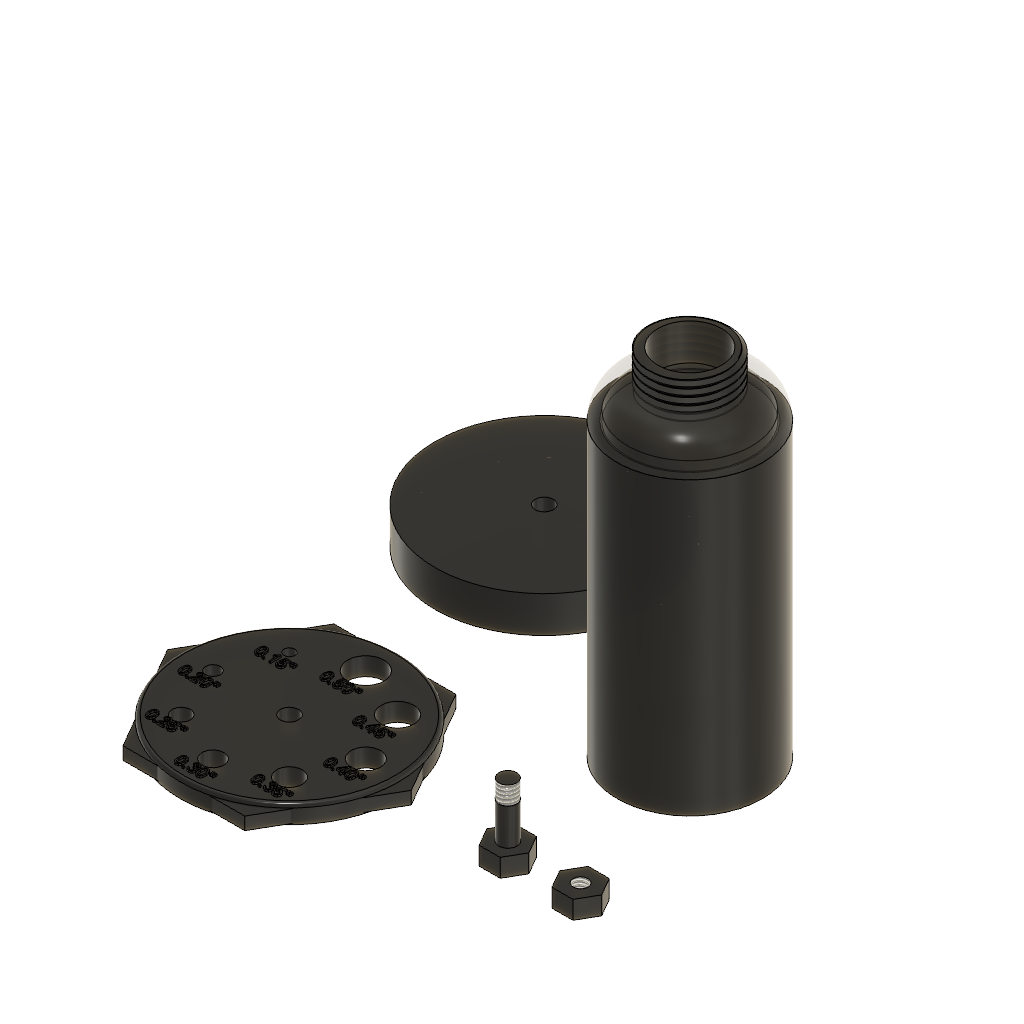
PillFilter Proof of Concept (Autodesk Fusion 360 design; units mm, degrees)
Autodesk Fusion 360 part; units mm, degrees
note: some values were not read from the file. Set by a fixed rule: the direction of a hole.
sketch "Filter Body" plane through (0, 0, 0) normal (0, 0, 1) x (1, 0, 0)
  circle A0 centre (0, 0) radius 38.1
  constraint coincident A0.centre origin
extrude "Extrude3" add sketch "Filter Body" along normal blind 6.35 makes body 1
hole "Hole5" at (0, 0, 6.35) direction (0, 0, -1) diameter 6.35 end through all bodies 1
sketch ".5\" Hole" plane through (0, 0, 6.35) normal (0, 0, 1) x (-1, 0, 0)
  circle A0 centre (0, 0) radius 3.175
  circle A1 centre (0, 0) radius 38.1
  circle A2 centre (0, -26.67) radius 6.35
  dimension "d27" = 12.7
  measures "d27" diameter of A2
sketch ".45\" Hole" plane through (0, 0, 6.35) normal (0, 0, 1) x (-1, 0, 0)
  circle A0 centre (-18.8585, -18.8585) radius 5.715
  dimension "d28" = 11.43
  measures "d28" diameter of A0
sketch ".4\" Hole" plane through (0, 0, 6.35) normal (0, 0, 1) x (-1, 0, 0)
  circle A0 centre (-26.67, 0) radius 5.08
  dimension "d29" = 10.16
  measures "d29" diameter of A0
sketch ".35\" Hole" plane through (0, 0, 6.35) normal (0, 0, 1) x (-1, 0, 0)
  circle A0 centre (-18.8585, 18.8585) radius 4.445
  dimension "d30" = 8.89
  measures "d30" diameter of A0
sketch "Lines (1.05\")" plane through (0, 0, 6.35) normal (0, 0, 1) x (1, 0, 0)
  line L0 (0, 0) -> (18.8585, 18.8585)
  line L1 (0, 0) -> (26.67, 0) construction
  line L2 (0, 0) -> (18.8585, -18.8585)
  line L3 (0, 0) -> (26.67, 0) construction
  line L4 (0, 0) -> (-18.8585, 18.8585)
  line L5 (0, 0) -> (-18.8585, -18.8585)
  line L6 (0, 0) -> (0, -26.67)
  line L7 (0, 0) -> (-26.67, 0)
  line L8 (0, 0) -> (0, 26.67)
  dimension "d31" = 45
  dimension "d32" = 26.67
  dimension "d33" = 45
  dimension "d34" = 26.67
  dimension "d36" = 26.67
  dimension "d37" = 26.67
  dimension "d38" = 26.67
  dimension "d39" = 26.67
  dimension "d45" = 26.67
  constraint horizontal L1
  constraint coincident L0.start L1.start
  constraint horizontal L3
  constraint perpendicular L0 L4
  constraint perpendicular L4 L5
  constraint perpendicular L1 L6
  constraint perpendicular L6 L7
  constraint perpendicular L3 L8
  measures "d31" angle of L0 L1
  measures "d32" distance of L0.start L0.end
  measures "d33" angle of L2 L3
  measures "d34" distance of L0.start L2.end
  measures "d36" distance of L0.start L4.end
  measures "d37" distance of L0.start L5.end
  measures "d38" distance of L0.start L6.end
  measures "d39" distance of L0.start L7.end
  measures "d45" distance of L0.start L8.end
sketch ".3\" Hole" plane through (0, 0, 6.35) normal (0, 0, 1) x (-1, 0, 0)
  circle A0 centre (0, 26.67) radius 3.81
  dimension "d41" = 7.62
  measures "d41" diameter of A0
sketch ".25\" Hole" plane through (0, 0, 6.35) normal (0, 0, 1) x (-1, 0, 0)
  circle A0 centre (18.8585, 18.8585) radius 3.175
  dimension "d42" = 6.35
  measures "d42" diameter of A0
sketch ".2\" Hole" plane through (0, 0, 6.35) normal (0, 0, 1) x (-1, 0, 0)
  circle A0 centre (26.67, 0) radius 2.54
  dimension "d43" = 5.08
  measures "d43" diameter of A0
sketch ".15\" Hole" plane through (0, 0, 6.35) normal (0, 0, 1) x (-1, 0, 0)
  circle A0 centre (18.8585, -18.8585) radius 1.905
  dimension "d44" = 3.81
  measures "d44" diameter of A0
hole "Hole6" at (0, 26.67, 6.35) direction (0, 0, -1) diameter 12.7 end through all bodies 1
hole "Hole7" at (18.8585, 18.8585, 6.35) direction (0, 0, -1) diameter 11.43 depth 12.7 tip angle 118 bodies 1
hole "Hole8" at (26.67, 0, 6.35) direction (0, 0, -1) diameter 10.16 end through all bodies 1
hole "Hole9" at (18.8585, -18.8585, 6.35) direction (0, 0, -1) diameter 8.89 depth 6.35 tip angle 118 bodies 1
hole "Hole10" at (0, -26.67, 6.35) direction (0, 0, -1) diameter 7.62 depth 6.35 tip angle 118 bodies 1
hole "Hole11" at (-18.8585, -18.8585, 6.35) direction (0, 0, -1) diameter 6.35 depth 6.35 tip angle 118 bodies 1
hole "Hole12" at (-26.67, 0, 6.35) direction (0, 0, -1) diameter 5.08 depth 6.35 tip angle 118 bodies 1
hole "Hole13" at (-18.8585, 18.8585, 6.35) direction (0, 0, -1) diameter 3.81 end through all bodies 1
sketch "Filter Backplate" plane through (0, 0, 0) normal (0, 0, 1) x (1, 0, 0)
  circle A0 centre (0, 88.9) radius 38.1
extrude "Extrude4" add sketch "Filter Backplate" along normal blind 6.35 separate body makes body 2
sketch "Backplate .5\" Hole" plane through (0, 0, 0) normal (0, 0, 1) x (1, 0, 0)
  circle A0 centre (0, 115.57) radius 6.35
  dimension "d71" = 12.7
  measures "d71" diameter of A0
hole "Hole14" at (0, 115.57, 0) direction (0, 0, 1) diameter 12.7 depth 12.7 tip angle 118 bodies 2
hole "Hole15" at (0, 88.9, 6.35) direction (0, 0, -1) diameter 6.35 end through all bodies 2
sketch "\"Text" plane through (0, 0, 6.35) normal (0, 0, 1) x (-1, 0, 0)
  line L0 (5.08, -16.51) -> (-5.08, -16.51) construction
  line L1 (-5.08, -16.51) -> (-5.08, -19.05) construction
  line L2 (-5.08, -19.05) -> (5.08, -19.05) construction
  line L3 (5.08, -19.05) -> (5.08, -16.51) construction
  line L4 (-15.2738, -8.7841) -> (-22.8759, -8.929) construction
  line L5 (-22.8759, -8.929) -> (-22.8262, -11.5359) construction
  line L6 (-22.8262, -11.5359) -> (-15.2241, -11.391) construction
  line L7 (-15.2241, -11.391) -> (-15.2738, -8.7841) construction
  line L8 (-22.86, 8.89) -> (-30.48, 8.89) construction
  line L9 (-30.48, 8.89) -> (-30.48, 6.35) construction
  line L10 (-30.48, 6.35) -> (-22.86, 6.35) construction
  line L11 (-22.86, 6.35) -> (-22.86, 8.89) construction
  line L12 (-15.24, 26.67) -> (-22.86, 26.67) construction
  line L13 (-22.86, 26.67) -> (-22.86, 24.13) construction
  line L14 (-22.86, 24.13) -> (-15.24, 24.13) construction
  line L15 (-15.24, 24.13) -> (-15.24, 26.67) construction
  line L16 (5.08, 34.29) -> (-5.08, 34.29) construction
  line L17 (-5.08, 34.29) -> (-5.08, 31.75) construction
  line L18 (-5.08, 31.75) -> (5.08, 31.75) construction
  line L19 (5.08, 31.75) -> (5.08, 34.29) construction
  line L20 (22.86, 25.4) -> (15.24, 25.4) construction
  line L21 (15.24, 25.4) -> (15.24, 22.86) construction
  line L22 (15.24, 22.86) -> (22.86, 22.86) construction
  line L23 (22.86, 22.86) -> (22.86, 25.4) construction
  line L24 (30.48, 6.35) -> (22.86, 6.35) construction
  line L25 (22.86, 6.35) -> (22.86, 3.81) construction
  line L26 (22.86, 3.81) -> (30.48, 3.81) construction
  line L27 (30.48, 3.81) -> (30.48, 6.35) construction
  line L28 (22.86, -12.7) -> (15.24, -12.7) construction
  line L29 (15.24, -12.7) -> (15.24, -15.24) construction
  line L30 (15.24, -15.24) -> (22.86, -15.24) construction
  line L31 (22.86, -15.24) -> (22.86, -12.7) construction
  dimension "d77" = 3.81
  dimension "d78" = 0
  dimension "d79" = 3.81
  dimension "d80" = 0
  dimension "d81" = 3.81
  dimension "d82" = 0
  dimension "d83" = 3.81
  dimension "d84" = 0
  dimension "d85" = 3.81
  dimension "d86" = 0
  dimension "d87" = 3.81
  dimension "d88" = 0
  dimension "d89" = 3.81
  dimension "d90" = 0
  dimension "d91" = 3.81
  dimension "d92" = 0
  text T0 "0.50\"" font "Arial" height 3.81 align centre middle in box 10.16 x 2.54 at (5.08, -16.51) x (-1, 0) y (0, -1) spacing 1 kerned
  text T1 "0.45\"" font "Arial" height 3.81 align centre middle in box 7.6035 x 2.6074 at (-15.2738, -8.7841) x (-0.999818, -0.019056) y (0.019056, -0.999818) spacing 1 kerned
  text T2 "0.40\"" font "Arial" height 3.81 align centre middle in box 7.62 x 2.54 at (-22.86, 8.89) x (-1, 0) y (0, -1) spacing 1 kerned
  text T3 "0.35\"" font "Arial" height 3.81 align centre middle in box 7.62 x 2.54 at (-15.24, 26.67) x (-1, 0) y (0, -1) spacing 1 kerned
  text T4 "0.30\"" font "Arial" height 3.81 align centre middle in box 10.16 x 2.54 at (5.08, 34.29) x (-1, 0) y (0, -1) spacing 1 kerned
  text T5 "0.25\"" font "Arial" height 3.81 align centre middle in box 7.62 x 2.54 at (22.86, 25.4) x (-1, 0) y (0, -1) spacing 1 kerned
  text T6 "0.20\"" font "Arial" height 3.81 align centre middle in box 7.62 x 2.54 at (30.48, 6.35) x (-1, 0) y (0, -1) spacing 1 kerned
  text T7 "0.15\"" font "Arial" height 3.81 align centre middle in box 7.62 x 2.54 at (22.86, -12.7) x (-1, 0) y (0, -1) spacing 1 kerned
extrude "Extrude5" add sketch "\"Text" along normal blind 0.635 text T0 T1 T2 T3 T4 T5 T6 T7 bodies 1
fillet "Fillet1" radius 1.27 1 edges at (-35.5217, -13.7775, 6.35) on bodies 1
sketch "Hex-Grip" plane through (0, 0, 0) normal (0, 0, 1) x (1, 0, 0)
  line L0 (-21.2638, 36.83) -> (-42.5276, 0)
  line L1 (-42.5276, 0) -> (-21.2638, -36.83)
  line L2 (-21.2638, -36.83) -> (21.2638, -36.83)
  line L3 (21.2638, -36.83) -> (42.5276, 0)
  line L4 (42.5276, 0) -> (21.2638, 36.83)
  line L5 (21.2638, 36.83) -> (-21.2638, 36.83)
  dimension "d97" = 36.83
  measures "d97" distance of origin L5
extrude "Extrude6" add sketch "Hex-Grip" along normal blind 4.445 separate body makes body 3
move_body "Move1" bodies 3 to x (1, 0, 0) y (0, 1, 0) z (0, 0, 1) at (0, 0, 0.3175)
sketch "Sketch24" plane through (0, 0, 4.7625) normal (0, 0, 1) x (-1, 0, 0)
  line L0 (-21.2638, -36.83) -> (21.2638, -36.83)
  line L1 (21.2638, -36.83) -> (42.5276, 0)
  line L2 (42.5276, 0) -> (21.2638, 36.83)
  line L3 (21.2638, 36.83) -> (-21.2638, 36.83)
  line L4 (-21.2638, 36.83) -> (-42.5276, 0)
  line L5 (-42.5276, 0) -> (-21.2638, -36.83)
hole "Hole16" at (0, 0, 4.7625) direction (0, 0, -1) diameter 67.31 depth 15.24 tip angle 118 bodies 3
sketch "Neck" plane through (0, 0, 0) normal (0, 0, -1) x (1, 0, 0)
  circle A0 centre (0, -88.9) radius 3.175
  circle A1 centre (0, -115.57) radius 6.35
  circle A2 centre (0, -88.9) radius 38.1
  circle A3 centre (0, -111.125) radius 15.875
  dimension "d103" = 31.75
  measures "d103" diameter of A3
extrude "Extrude7" add sketch "Neck" along normal blind 12.7 contours A3 bodies 2
move_body "Move2" bodies 2 to x (1, 0, 0) y (0, 1, 0) z (0, 0, 1) at (0, 0, 12.7)
sketch "Neck Receptacle" plane through (0, 0, 0) normal (0, 0, -1) x (1, 0, 0)
  circle A0 centre (0, -111.125) radius 13.335
hole "Hole17" at (0, 111.125, 0) direction (0, 0, 1) diameter 25.4 depth 12.7 tip angle 180 bodies 2
thread "Thread1" "ANSI Unified Screw Threads 1.125 1 1/8-10 UNS 1 1/8-10 UNS 2B" major diameter 28.575 minor diameter 26.0985 pitch 2.54 angle 60 modelled right hand crest width 0.7347 on face at (1.2645, 123.7619, 4.2333) crest through (-13.0493, 111.125, 0.635) on bodies 2
sketch "BottleBase" plane through (0, 0, 0) normal (0, 0, 1) x (1, 0, 0)
  circle A0 centre (76.2, 63.5) radius 25.4
  dimension "d111" = 50.8
  measures "d111" diameter of A0
extrude "Extrude8" add sketch "BottleBase" along normal blind 101.6 separate body makes body 4
hole "Hole18" at (76.2, 63.5, 101.6) direction (0, 0, -1) diameter 44.45 depth 98.425 tip angle 180 bodies 4
sketch "BottleShoulders" plane through (0, 0, 101.6) normal (0, 0, 1) x (-1, 0, 0)
  circle A0 centre (-76.2, -63.5) radius 22.225
  circle A1 centre (-76.2, -63.5) radius 25.4
  circle A2 centre (-76.2, -63.5) radius 25.4
  constraint concentric A0 A2
sketch "BottleShoulders (1)" plane through (0, 0, 101.6) normal (0, 0, 1) x (-1, 0, 0)
  circle A0 centre (-76.2, -63.5) radius 22.225
  circle A1 centre (-76.2, -63.5) radius 25.4
  circle A2 centre (-76.2, -63.5) radius 25.4
  constraint concentric A0 A2
extrude "Extrude10" add sketch "BottleShoulders (1)" along normal blind 12.7 separate body contours A0 | A1 A2 makes body 5
fillet "Fillet2" radius 12.7 1 edges at (99.8811, 72.685, 114.3) on bodies 5
shell "Shell1" thickness 3.175 removed faces 0 bodies 5
hole "Hole19" at (76.2, 63.5, 114.3) direction (0, 0, -1) diameter 25.4 depth 25.4 tip angle 180 bodies 5
hole "Hole20" at (76.2, 63.5, 104.775) direction (0, 0, -1) diameter 43.434 depth 25.4 tip angle 180 bodies 5
sketch "BottleNeck" plane through (0, 0, 101.6) normal (0, 0, 1) x (-1, 0, 0)
  circle A0 centre (-76.2, -63.5) radius 22.225
  circle A1 centre (-76.2, -63.5) radius 25.4
  circle A2 centre (-76.2, -63.5) radius 12.7
  dimension "d130" = 25.4
  constraint concentric A0 A2
  measures "d130" diameter of A2
extrude "Extrude11" add sketch "BottleNeck" along normal blind 12.7 separate body contours A2 makes body 6
move_body "Move3" bodies 6 to x (1, 0, 0) y (0, 1, 0) z (0, 0, 1) at (0, 0, 17.78)
move_body "Move4" bodies 6 to x (1, 0, 0) y (0, 1, 0) z (0, 0, 1) at (0, 0, -8.255)
thread "Thread2" "ANSI Unified Screw Threads 1.125 1 1/8-10 UNS 1 1/8-10 UNS 2A" major diameter 28.3667 minor diameter 25.5067 pitch 2.54 angle 60 modelled right hand crest width 0.3652 on face at (63.5631, 64.7645, 119.5917) crest through (62.0166, 63.5, 110.49) on bodies 6
hole "Hole21" at (76.2, 63.5, 123.825) direction (0, 0, -1) diameter 22.225 depth 25.4 tip angle 180 bodies 6
extrude "Extrude12" add 1 faces at (-13.0647, 104.1536, 19.05) along direction (0, 0, 1) blind 6.35 on bodies 2 bodies 2
sketch "BoltHead" plane through (0, 0, 0) normal (0, 0, 1) x (1, 0, 0)
  line L0 (72.5338, 6.35) -> (68.8677, 0)
  line L1 (68.8677, 0) -> (72.5338, -6.35)
  line L2 (72.5338, -6.35) -> (79.8662, -6.35)
  line L3 (79.8662, -6.35) -> (83.5324, 0)
  line L4 (83.5324, 0) -> (79.8662, 6.35)
  line L5 (79.8662, 6.35) -> (72.5338, 6.35)
  point P0 (76.2, 0)
  dimension "d146" = 6.35
  measures "d146" distance of P0 L5
extrude "Extrude13" add sketch "BoltHead" along normal blind 6.35 separate body makes body 7
sketch "BoltShank" plane through (0, 0, 6.35) normal (0, 0, 1) x (-1, 0, 0)
  line L0 (-79.8662, -6.35) -> (-72.5338, -6.35)
  line L1 (-72.5338, -6.35) -> (-68.8677, 0)
  line L2 (-68.8677, 0) -> (-72.5338, 6.35)
  line L3 (-72.5338, 6.35) -> (-79.8662, 6.35)
  line L4 (-79.8662, 6.35) -> (-83.5324, 0)
  line L5 (-83.5324, 0) -> (-79.8662, -6.35)
  circle A0 centre (-76.2, 0) radius 3.175
  dimension "d149" = 6.35
  measures "d149" diameter of A0
extrude "Extrude14" add sketch "BoltShank" along normal blind 12.7 contours A0 bodies 7
extrude "Extrude15" add 1 faces at (75.1887, 0.3119, 19.05) along direction (0, 0, 1) blind 6.35 separate body on bodies 7 makes body 8
thread "Thread3" "ANSI Unified Screw Threads 0.25 1/4-20 UNC 1/4-20 UNC 3A" major diameter 6.2484 minor diameter 4.8387 pitch 1.27 angle 60 resizes the face on face at (73.0408, 0.3161, 23.2833) on bodies 8
sketch "Nut" plane through (0, 0, 0) normal (0, 0, 1) x (1, 0, 0)
  line L0 (97.9338, 6.35) -> (94.2677, 0)
  line L1 (94.2677, 0) -> (97.9338, -6.35)
  line L2 (97.9338, -6.35) -> (105.2662, -6.35)
  line L3 (105.2662, -6.35) -> (108.9324, 0)
  line L4 (108.9324, 0) -> (105.2662, 6.35)
  line L5 (105.2662, 6.35) -> (97.9338, 6.35)
  point P0 (101.6, 0)
  dimension "d156" = 6.35
  measures "d156" distance of P0 L5
extrude "Extrude16" add sketch "Nut" along normal blind 6.35 separate body makes body 9
hole "Hole22" at (101.6, 0, 6.35) direction (0, 0, -1) diameter 6.35 depth 6.35 tip angle 180 bodies 9
thread "Thread4" "ANSI Unified Screw Threads 0.25 1/4-20 UNC 1/4-20 UNC 3B" major diameter 6.35 minor diameter 5.1156 pitch 1.27 angle 60 resizes the face on face at (100.8165, -3.0768, 4.2333) on bodies 9
equation "d78 = '0.50\"'"
equation "d80 = '0.45\"'"
equation "d82 = '0.40\"'"
equation "d84 = '0.35\"'"
equation "d86 = '0.30\"'"
equation "d88 = '0.25\"'"
equation "d90 = '0.20\"'"
equation "d92 = '0.15\"'"
named bodies: "Filter body", "Filter Backplate", "Hex Grip", "Bottle", "Bottle Shoulders", "Bottle Neck", "Bolt Head/Shank", "BoltThread", "Nut"
